Autodesk Fusion 360 part; units mm, degrees
(part 2 of 5)
sketch "Clamp Features" plane through (0, 0, 0) normal (0, 0, 1) x (1, 0, 0) in component "SpoilBoard"
  line L0 (576.58, 93.1525) -> (642.62, 93.1525)
  arc A0 (642.62, 93.1525) -> (642.62, 133.1525) centre (642.62, 113.1525) ccw
  line L1 (642.62, 133.1525) -> (576.58, 133.1525)
  arc A1 (576.58, 133.1525) -> (576.58, 93.1525) centre (576.58, 113.1525) ccw
  line L2 (576.58, 113.1525) -> (642.62, 113.1525) construction
  line L3 (0, 0) -> (1219.2, 0)
  line L4 (609.6, 0) -> (609.6, 113.1525)
  line L5 (33.02, 93.1525) -> (99.06, 93.1525)
  line L6 (99.06, 133.1525) -> (33.02, 133.1525)
  line L7 (33.02, 113.1525) -> (99.06, 113.1525) construction
  arc A2 (99.06, 93.1525) -> (99.06, 133.1525) centre (99.06, 113.1525) ccw
  arc A3 (33.02, 133.1525) -> (33.02, 93.1525) centre (33.02, 113.1525) ccw
  line L8 (214.2067, 93.1525) -> (280.2467, 93.1525)
  line L9 (280.2467, 133.1525) -> (214.2067, 133.1525)
  line L10 (214.2067, 113.1525) -> (280.2467, 113.1525) construction
  arc A4 (280.2467, 93.1525) -> (280.2467, 133.1525) centre (280.2467, 113.1525) ccw
  arc A5 (214.2067, 133.1525) -> (214.2067, 93.1525) centre (214.2067, 113.1525) ccw
  line L11 (395.3933, 93.1525) -> (461.4333, 93.1525)
  line L12 (461.4333, 133.1525) -> (395.3933, 133.1525)
  line L13 (395.3933, 113.1525) -> (461.4333, 113.1525) construction
  arc A6 (461.4333, 93.1525) -> (461.4333, 133.1525) centre (461.4333, 113.1525) ccw
  arc A7 (395.3933, 133.1525) -> (395.3933, 93.1525) centre (395.3933, 113.1525) ccw
  line L14 (757.7667, 93.1525) -> (823.8067, 93.1525)
  line L15 (823.8067, 133.1525) -> (757.7667, 133.1525)
  line L16 (757.7667, 113.1525) -> (823.8067, 113.1525) construction
  arc A8 (823.8067, 93.1525) -> (823.8067, 133.1525) centre (823.8067, 113.1525) ccw
  arc A9 (757.7667, 133.1525) -> (757.7667, 93.1525) centre (757.7667, 113.1525) ccw
  line L17 (938.9533, 93.1525) -> (1004.9933, 93.1525)
  line L18 (1004.9933, 133.1525) -> (938.9533, 133.1525)
  line L19 (938.9533, 113.1525) -> (1004.9933, 113.1525) construction
  arc A10 (1004.9933, 93.1525) -> (1004.9933, 133.1525) centre (1004.9933, 113.1525) ccw
  arc A11 (938.9533, 133.1525) -> (938.9533, 93.1525) centre (938.9533, 113.1525) ccw
  line L20 (1120.14, 93.1525) -> (1186.18, 93.1525)
  line L21 (1186.18, 133.1525) -> (1120.14, 133.1525)
  line L22 (1120.14, 113.1525) -> (1186.18, 113.1525) construction
  arc A12 (1186.18, 93.1525) -> (1186.18, 133.1525) centre (1186.18, 113.1525) ccw
  arc A13 (1120.14, 133.1525) -> (1120.14, 93.1525) centre (1120.14, 113.1525) ccw
  line L23 (33.02, 313.1525) -> (99.06, 313.1525)
  line L24 (99.06, 353.1525) -> (33.02, 353.1525)
  line L25 (33.02, 333.1525) -> (99.06, 333.1525) construction
  arc A14 (99.06, 313.1525) -> (99.06, 353.1525) centre (99.06, 333.1525) ccw
  arc A15 (33.02, 353.1525) -> (33.02, 313.1525) centre (33.02, 333.1525) ccw
  line L26 (214.2067, 313.1525) -> (280.2467, 313.1525)
  line L27 (280.2467, 353.1525) -> (214.2067, 353.1525)
  line L28 (214.2067, 333.1525) -> (280.2467, 333.1525) construction
  arc A16 (280.2467, 313.1525) -> (280.2467, 353.1525) centre (280.2467, 333.1525) ccw
  arc A17 (214.2067, 353.1525) -> (214.2067, 313.1525) centre (214.2067, 333.1525) ccw
  line L29 (395.3933, 313.1525) -> (461.4333, 313.1525)
  line L30 (461.4333, 353.1525) -> (395.3933, 353.1525)
  line L31 (395.3933, 333.1525) -> (461.4333, 333.1525) construction
  arc A18 (461.4333, 313.1525) -> (461.4333, 353.1525) centre (461.4333, 333.1525) ccw
  arc A19 (395.3933, 353.1525) -> (395.3933, 313.1525) centre (395.3933, 333.1525) ccw
  line L32 (576.58, 313.1525) -> (642.62, 313.1525)
  line L33 (642.62, 353.1525) -> (576.58, 353.1525)
  line L34 (576.58, 333.1525) -> (642.62, 333.1525) construction
  arc A20 (642.62, 313.1525) -> (642.62, 353.1525) centre (642.62, 333.1525) ccw
  arc A21 (576.58, 353.1525) -> (576.58, 313.1525) centre (576.58, 333.1525) ccw
  line L35 (757.7667, 313.1525) -> (823.8067, 313.1525)
  line L36 (823.8067, 353.1525) -> (757.7667, 353.1525)
  line L37 (757.7667, 333.1525) -> (823.8067, 333.1525) construction
  arc A22 (823.8067, 313.1525) -> (823.8067, 353.1525) centre (823.8067, 333.1525) ccw
  arc A23 (757.7667, 353.1525) -> (757.7667, 313.1525) centre (757.7667, 333.1525) ccw
  line L38 (938.9533, 313.1525) -> (1004.9933, 313.1525)
  line L39 (1004.9933, 353.1525) -> (938.9533, 353.1525)
  line L40 (938.9533, 333.1525) -> (1004.9933, 333.1525) construction
  arc A24 (1004.9933, 313.1525) -> (1004.9933, 353.1525) centre (1004.9933, 333.1525) ccw
  arc A25 (938.9533, 353.1525) -> (938.9533, 313.1525) centre (938.9533, 333.1525) ccw
  line L41 (1120.14, 313.1525) -> (1186.18, 313.1525)
  line L42 (1186.18, 353.1525) -> (1120.14, 353.1525)
  line L43 (1120.14, 333.1525) -> (1186.18, 333.1525) construction
  arc A26 (1186.18, 313.1525) -> (1186.18, 353.1525) centre (1186.18, 333.1525) ccw
  arc A27 (1120.14, 353.1525) -> (1120.14, 313.1525) centre (1120.14, 333.1525) ccw
  line L44 (665.5361, 207.1642) -> (731.5761, 207.1637)
  arc A28 (731.5761, 207.1637) -> (731.5763, 247.1637) centre (731.5762, 227.1637) ccw
  line L45 (665.5362, 227.1642) -> (731.5762, 227.1637) construction
  arc A29 (666.0507, 247.1575) -> (665.5361, 207.1642) centre (666.0526, 227.1575) ccw
  line L46 (731.5763, 247.1637) -> (666.0507, 247.1575)
  line L47 (666.0526, 227.1575) -> (731.1, 227.1575) construction
  line L48 (487.6237, 247.1637) -> (553.1493, 247.1575)
  arc A30 (553.6639, 207.1642) -> (553.1493, 247.1575) centre (553.1474, 227.1575) ccw
  line L49 (553.6639, 207.1642) -> (487.6239, 207.1637)
  arc A31 (487.6237, 247.1637) -> (487.6239, 207.1637) centre (487.6238, 227.1637) ccw
  line L50 (553.6638, 227.1642) -> (487.6238, 227.1637) construction
  line L51 (851.0526, 227.1575) -> (916.1, 227.1575) construction
  arc A32 (851.0507, 247.1575) -> (850.5361, 207.1642) centre (851.0526, 227.1575) ccw
  line L52 (850.5361, 207.1642) -> (916.5761, 207.1637)
  line L53 (916.5763, 247.1637) -> (851.0507, 247.1575)
  arc A33 (916.5761, 207.1637) -> (916.5763, 247.1637) centre (916.5762, 227.1637) ccw
  line L54 (850.5362, 227.1642) -> (916.5762, 227.1637) construction
  line L55 (1036.0526, 227.1575) -> (1101.1, 227.1575) construction
  arc A34 (1036.0507, 247.1575) -> (1035.5361, 207.1642) centre (1036.0526, 227.1575) ccw
  line L56 (1035.5361, 207.1642) -> (1101.5761, 207.1637)
  line L57 (1101.5763, 247.1637) -> (1036.0507, 247.1575)
  arc A35 (1101.5761, 207.1637) -> (1101.5763, 247.1637) centre (1101.5762, 227.1637) ccw
  line L58 (1035.5362, 227.1642) -> (1101.5762, 227.1637) construction
  line L59 (368.6639, 207.1642) -> (302.6239, 207.1637)
  arc A36 (368.6639, 207.1642) -> (368.1493, 247.1575) centre (368.1474, 227.1575) ccw
  line L60 (302.6237, 247.1637) -> (368.1493, 247.1575)
  arc A37 (302.6237, 247.1637) -> (302.6239, 207.1637) centre (302.6238, 227.1637) ccw
  line L61 (183.6639, 207.1642) -> (117.6239, 207.1637)
  arc A38 (183.6639, 207.1642) -> (183.1493, 247.1575) centre (183.1474, 227.1575) ccw
  line L62 (117.6237, 247.1637) -> (183.1493, 247.1575)
  arc A39 (117.6237, 247.1637) -> (117.6239, 207.1637) centre (117.6238, 227.1637) ccw
  line L63 (33.02, 713.1525) -> (99.06, 713.1525)
  arc A40 (461.4333, 713.1525) -> (461.4333, 753.1525) centre (461.4333, 733.1525) ccw
  arc A41 (395.3933, 753.1525) -> (395.3933, 713.1525) centre (395.3933, 733.1525) ccw
  line L64 (99.06, 753.1525) -> (33.02, 753.1525)
  arc A42 (576.58, 753.1525) -> (576.58, 713.1525) centre (576.58, 733.1525) ccw
  line L65 (33.02, 733.1525) -> (99.06, 733.1525) construction
  line L66 (214.2067, 713.1525) -> (280.2467, 713.1525)
  arc A43 (214.2067, 753.1525) -> (214.2067, 713.1525) centre (214.2067, 733.1525) ccw
  arc A44 (280.2467, 713.1525) -> (280.2467, 753.1525) centre (280.2467, 733.1525) ccw
  line L67 (280.2467, 753.1525) -> (214.2067, 753.1525)
  arc A45 (1120.14, 753.1525) -> (1120.14, 713.1525) centre (1120.14, 733.1525) ccw
  line L68 (938.9533, 733.1525) -> (1004.9933, 733.1525) construction
  line L69 (1120.14, 713.1525) -> (1186.18, 713.1525)
  line L70 (1186.18, 753.1525) -> (1120.14, 753.1525)
  line L71 (1120.14, 733.1525) -> (1186.18, 733.1525) construction
  arc A46 (1004.9933, 713.1525) -> (1004.9933, 753.1525) centre (1004.9933, 733.1525) ccw
  arc A47 (1186.18, 713.1525) -> (1186.18, 753.1525) centre (1186.18, 733.1525) ccw
  arc A48 (33.02, 753.1525) -> (33.02, 713.1525) centre (33.02, 733.1525) ccw
  line L72 (214.2067, 733.1525) -> (280.2467, 733.1525) construction
  arc A49 (99.06, 713.1525) -> (99.06, 753.1525) centre (99.06, 733.1525) ccw
  arc A50 (642.62, 713.1525) -> (642.62, 753.1525) centre (642.62, 733.1525) ccw
  arc A51 (823.8067, 713.1525) -> (823.8067, 753.1525) centre (823.8067, 733.1525) ccw
  arc A52 (938.9533, 753.1525) -> (938.9533, 713.1525) centre (938.9533, 733.1525) ccw
  line L73 (938.9533, 713.1525) -> (1004.9933, 713.1525)
  line L74 (1004.9933, 753.1525) -> (938.9533, 753.1525)
  line L75 (757.7667, 713.1525) -> (823.8067, 713.1525)
  line L76 (823.8067, 753.1525) -> (757.7667, 753.1525)
  line L77 (757.7667, 733.1525) -> (823.8067, 733.1525) construction
  arc A53 (757.7667, 753.1525) -> (757.7667, 713.1525) centre (757.7667, 733.1525) ccw
  line L78 (395.3933, 713.1525) -> (461.4333, 713.1525)
  line L79 (461.4333, 753.1525) -> (395.3933, 753.1525)
  line L80 (395.3933, 733.1525) -> (461.4333, 733.1525) construction
  line L81 (576.58, 713.1525) -> (642.62, 713.1525)
  line L82 (642.62, 753.1525) -> (576.58, 753.1525)
  line L83 (576.58, 733.1525) -> (642.62, 733.1525) construction
  line L84 (665.5361, 607.1642) -> (731.5761, 607.1637)
  line L85 (666.0526, 627.1575) -> (731.1, 627.1575) construction
  line L86 (850.5361, 607.1642) -> (916.5761, 607.1637)
  line L87 (665.5362, 627.1642) -> (731.5762, 627.1637) construction
  arc A54 (851.0507, 647.1575) -> (850.5361, 607.1642) centre (851.0526, 627.1575) ccw
  line L88 (850.5362, 627.1642) -> (916.5762, 627.1637) construction
  line L89 (851.0526, 627.1575) -> (916.1, 627.1575) construction
  arc A55 (916.5761, 607.1637) -> (916.5763, 647.1637) centre (916.5762, 627.1637) ccw
  line L90 (916.5763, 647.1637) -> (851.0507, 647.1575)
  line L91 (731.5763, 647.1637) -> (666.0507, 647.1575)
  arc A56 (731.5761, 607.1637) -> (731.5763, 647.1637) centre (731.5762, 627.1637) ccw
  arc A57 (1101.5761, 607.1637) -> (1101.5763, 647.1637) centre (1101.5762, 627.1637) ccw
  arc A58 (368.6639, 607.1642) -> (368.1493, 647.1575) centre (368.1474, 627.1575) ccw
  line L92 (368.6639, 607.1642) -> (302.6239, 607.1637)
  line L93 (302.6237, 647.1637) -> (368.1493, 647.1575)
  line L94 (183.6639, 607.1642) -> (117.6239, 607.1637)
  line L95 (117.6237, 647.1637) -> (183.1493, 647.1575)
  arc A59 (302.6237, 647.1637) -> (302.6239, 607.1637) centre (302.6238, 627.1637) ccw
  arc A60 (183.6639, 607.1642) -> (183.1493, 647.1575) centre (183.1474, 627.1575) ccw
  arc A61 (117.6237, 647.1637) -> (117.6239, 607.1637) centre (117.6238, 627.1637) ccw
  line L96 (1035.5361, 607.1642) -> (1101.5761, 607.1637)
  line L97 (1101.5763, 647.1637) -> (1036.0507, 647.1575)
  line L98 (1035.5362, 627.1642) -> (1101.5762, 627.1637) construction
  arc A62 (1036.0507, 647.1575) -> (1035.5361, 607.1642) centre (1036.0526, 627.1575) ccw
  arc A63 (553.6639, 607.1642) -> (553.1493, 647.1575) centre (553.1474, 627.1575) ccw
  line L99 (553.6638, 627.1642) -> (487.6238, 627.1637) construction
  line L100 (553.6639, 607.1642) -> (487.6239, 607.1637)
  line L101 (487.6237, 647.1637) -> (553.1493, 647.1575)
  arc A64 (487.6237, 647.1637) -> (487.6239, 607.1637) centre (487.6238, 627.1637) ccw
  line L102 (1036.0526, 627.1575) -> (1101.1, 627.1575) construction
  arc A65 (666.0507, 647.1575) -> (665.5361, 607.1642) centre (666.0526, 627.1575) ccw
  line L103 (938.9533, 493.1525) -> (1004.9933, 493.1525)
  line L104 (1004.9933, 533.1525) -> (938.9533, 533.1525)
  line L105 (938.9533, 513.1525) -> (1004.9933, 513.1525) construction
  line L106 (1120.14, 493.1525) -> (1186.18, 493.1525)
  line L107 (1186.18, 533.1525) -> (1120.14, 533.1525)
  line L108 (1120.14, 513.1525) -> (1186.18, 513.1525) construction
  arc A66 (1004.9933, 493.1525) -> (1004.9933, 533.1525) centre (1004.9933, 513.1525) ccw
  arc A67 (1186.18, 493.1525) -> (1186.18, 533.1525) centre (1186.18, 513.1525) ccw
  arc A68 (1120.14, 533.1525) -> (1120.14, 493.1525) centre (1120.14, 513.1525) ccw
  line L109 (757.7667, 493.1525) -> (823.8067, 493.1525)
  line L110 (757.7667, 513.1525) -> (823.8067, 513.1525) construction
  line L111 (823.8067, 533.1525) -> (757.7667, 533.1525)
  arc A69 (823.8067, 493.1525) -> (823.8067, 533.1525) centre (823.8067, 513.1525) ccw
  arc A70 (938.9533, 533.1525) -> (938.9533, 493.1525) centre (938.9533, 513.1525) ccw
  arc A71 (642.62, 493.1525) -> (642.62, 533.1525) centre (642.62, 513.1525) ccw
  line L112 (33.02, 493.1525) -> (99.06, 493.1525)
  arc A72 (576.58, 533.1525) -> (576.58, 493.1525) centre (576.58, 513.1525) ccw
  line L113 (99.06, 533.1525) -> (33.02, 533.1525)
  arc A73 (33.02, 533.1525) -> (33.02, 493.1525) centre (33.02, 513.1525) ccw
  arc A74 (461.4333, 493.1525) -> (461.4333, 533.1525) centre (461.4333, 513.1525) ccw
  line L114 (33.02, 513.1525) -> (99.06, 513.1525) construction
  arc A75 (99.06, 493.1525) -> (99.06, 533.1525) centre (99.06, 513.1525) ccw
  arc A76 (395.3933, 533.1525) -> (395.3933, 493.1525) centre (395.3933, 513.1525) ccw
  line L115 (214.2067, 493.1525) -> (280.2467, 493.1525)
  line L116 (280.2467, 533.1525) -> (214.2067, 533.1525)
  line L117 (214.2067, 513.1525) -> (280.2467, 513.1525) construction
  arc A77 (757.7667, 533.1525) -> (757.7667, 493.1525) centre (757.7667, 513.1525) ccw
  arc A78 (214.2067, 533.1525) -> (214.2067, 493.1525) centre (214.2067, 513.1525) ccw
  line L118 (576.58, 493.1525) -> (642.62, 493.1525)
  line L119 (576.58, 513.1525) -> (642.62, 513.1525) construction
  line L120 (609.6, 400) -> (609.6, 513.1525)
  line L121 (395.3933, 493.1525) -> (461.4333, 493.1525)
  line L122 (395.3933, 513.1525) -> (461.4333, 513.1525) construction
  arc A79 (280.2467, 493.1525) -> (280.2467, 533.1525) centre (280.2467, 513.1525) ccw
  line L123 (461.4333, 533.1525) -> (395.3933, 533.1525)
  line L124 (642.62, 533.1525) -> (576.58, 533.1525)
  line L125 (33.02, 1113.1525) -> (99.06, 1113.1525)
  arc A80 (461.4333, 1113.1525) -> (461.4333, 1153.1525) centre (461.4333, 1133.1525) ccw
  arc A81 (395.3933, 1153.1525) -> (395.3933, 1113.1525) centre (395.3933, 1133.1525) ccw
  line L126 (99.06, 1153.1525) -> (33.02, 1153.1525)
  arc A82 (576.58, 1153.1525) -> (576.58, 1113.1525) centre (576.58, 1133.1525) ccw
  line L127 (33.02, 1133.1525) -> (99.06, 1133.1525) construction
  line L128 (214.2067, 1113.1525) -> (280.2467, 1113.1525)
  arc A83 (214.2067, 1153.1525) -> (214.2067, 1113.1525) centre (214.2067, 1133.1525) ccw
  arc A84 (280.2467, 1113.1525) -> (280.2467, 1153.1525) centre (280.2467, 1133.1525) ccw
  line L129 (280.2467, 1153.1525) -> (214.2067, 1153.1525)
  arc A85 (1120.14, 1153.1525) -> (1120.14, 1113.1525) centre (1120.14, 1133.1525) ccw
  line L130 (938.9533, 1133.1525) -> (1004.9933, 1133.1525) construction
  line L131 (1120.14, 1113.1525) -> (1186.18, 1113.1525)
  line L132 (1186.18, 1153.1525) -> (1120.14, 1153.1525)
  line L133 (1120.14, 1133.1525) -> (1186.18, 1133.1525) construction
  arc A86 (1004.9933, 1113.1525) -> (1004.9933, 1153.1525) centre (1004.9933, 1133.1525) ccw
  arc A87 (1186.18, 1113.1525) -> (1186.18, 1153.1525) centre (1186.18, 1133.1525) ccw
  arc A88 (33.02, 1153.1525) -> (33.02, 1113.1525) centre (33.02, 1133.1525) ccw
  line L134 (214.2067, 1133.1525) -> (280.2467, 1133.1525) construction
  arc A89 (99.06, 1113.1525) -> (99.06, 1153.1525) centre (99.06, 1133.1525) ccw
  arc A90 (642.62, 1113.1525) -> (642.62, 1153.1525) centre (642.62, 1133.1525) ccw
  arc A91 (823.8067, 1113.1525) -> (823.8067, 1153.1525) centre (823.8067, 1133.1525) ccw
  arc A92 (938.9533, 1153.1525) -> (938.9533, 1113.1525) centre (938.9533, 1133.1525) ccw
  line L135 (938.9533, 1113.1525) -> (1004.9933, 1113.1525)
  line L136 (1004.9933, 1153.1525) -> (938.9533, 1153.1525)
  line L137 (757.7667, 1113.1525) -> (823.8067, 1113.1525)
  line L138 (823.8067, 1153.1525) -> (757.7667, 1153.1525)
  line L139 (757.7667, 1133.1525) -> (823.8067, 1133.1525) construction
  arc A93 (757.7667, 1153.1525) -> (757.7667, 1113.1525) centre (757.7667, 1133.1525) ccw
  line L140 (395.3933, 1113.1525) -> (461.4333, 1113.1525)
  line L141 (461.4333, 1153.1525) -> (395.3933, 1153.1525)
  line L142 (395.3933, 1133.1525) -> (461.4333, 1133.1525) construction
  line L143 (576.58, 1113.1525) -> (642.62, 1113.1525)
  line L144 (642.62, 1153.1525) -> (576.58, 1153.1525)
  line L145 (576.58, 1133.1525) -> (642.62, 1133.1525) construction
  line L146 (665.5361, 1007.1642) -> (731.5761, 1007.1637)
  line L147 (666.0526, 1027.1575) -> (731.1, 1027.1575) construction
  line L148 (850.5361, 1007.1642) -> (916.5761, 1007.1637)
  line L149 (665.5362, 1027.1642) -> (731.5762, 1027.1637) construction
  arc A94 (851.0507, 1047.1575) -> (850.5361, 1007.1642) centre (851.0526, 1027.1575) ccw
  line L150 (850.5362, 1027.1642) -> (916.5762, 1027.1637) construction
  line L151 (851.0526, 1027.1575) -> (916.1, 1027.1575) construction
  arc A95 (916.5761, 1007.1637) -> (916.5763, 1047.1637) centre (916.5762, 1027.1637) ccw
  line L152 (916.5763, 1047.1637) -> (851.0507, 1047.1575)
  line L153 (731.5763, 1047.1637) -> (666.0507, 1047.1575)
  arc A96 (731.5761, 1007.1637) -> (731.5763, 1047.1637) centre (731.5762, 1027.1637) ccw
  arc A97 (1101.5761, 1007.1637) -> (1101.5763, 1047.1637) centre (1101.5762, 1027.1637) ccw
  arc A98 (368.6639, 1007.1642) -> (368.1493, 1047.1575) centre (368.1474, 1027.1575) ccw
  line L154 (368.6639, 1007.1642) -> (302.6239, 1007.1637)
  line L155 (302.6237, 1047.1637) -> (368.1493, 1047.1575)
  line L156 (183.6639, 1007.1642) -> (117.6239, 1007.1637)
  line L157 (117.6237, 1047.1637) -> (183.1493, 1047.1575)
  arc A99 (302.6237, 1047.1637) -> (302.6239, 1007.1637) centre (302.6238, 1027.1637) ccw
  arc A100 (183.6639, 1007.1642) -> (183.1493, 1047.1575) centre (183.1474, 1027.1575) ccw
  arc A101 (117.6237, 1047.1637) -> (117.6239, 1007.1637) centre (117.6238, 1027.1637) ccw
  line L158 (1035.5361, 1007.1642) -> (1101.5761, 1007.1637)
  line L159 (1101.5763, 1047.1637) -> (1036.0507, 1047.1575)
  line L160 (1035.5362, 1027.1642) -> (1101.5762, 1027.1637) construction
  arc A102 (1036.0507, 1047.1575) -> (1035.5361, 1007.1642) centre (1036.0526, 1027.1575) ccw
  arc A103 (553.6639, 1007.1642) -> (553.1493, 1047.1575) centre (553.1474, 1027.1575) ccw
  line L161 (553.6638, 1027.1642) -> (487.6238, 1027.1637) construction
  line L162 (553.6639, 1007.1642) -> (487.6239, 1007.1637)
  line L163 (487.6237, 1047.1637) -> (553.1493, 1047.1575)
  arc A104 (487.6237, 1047.1637) -> (487.6239, 1007.1637) centre (487.6238, 1027.1637) ccw
  line L164 (1036.0526, 1027.1575) -> (1101.1, 1027.1575) construction
  arc A105 (666.0507, 1047.1575) -> (665.5361, 1007.1642) centre (666.0526, 1027.1575) ccw
  line L165 (938.9533, 893.1525) -> (1004.9933, 893.1525)
  line L166 (1004.9933, 933.1525) -> (938.9533, 933.1525)
  line L167 (938.9533, 913.1525) -> (1004.9933, 913.1525) construction
  line L168 (1120.14, 893.1525) -> (1186.18, 893.1525)
  line L169 (1186.18, 933.1525) -> (1120.14, 933.1525)
  line L170 (1120.14, 913.1525) -> (1186.18, 913.1525) construction
  arc A106 (1004.9933, 893.1525) -> (1004.9933, 933.1525) centre (1004.9933, 913.1525) ccw
  arc A107 (1186.18, 893.1525) -> (1186.18, 933.1525) centre (1186.18, 913.1525) ccw
  arc A108 (1120.14, 933.1525) -> (1120.14, 893.1525) centre (1120.14, 913.1525) ccw
  line L171 (757.7667, 893.1525) -> (823.8067, 893.1525)
  line L172 (757.7667, 913.1525) -> (823.8067, 913.1525) construction
  line L173 (823.8067, 933.1525) -> (757.7667, 933.1525)
  arc A109 (823.8067, 893.1525) -> (823.8067, 933.1525) centre (823.8067, 913.1525) ccw
  arc A110 (938.9533, 933.1525) -> (938.9533, 893.1525) centre (938.9533, 913.1525) ccw
  arc A111 (642.62, 893.1525) -> (642.62, 933.1525) centre (642.62, 913.1525) ccw
  line L174 (33.02, 893.1525) -> (99.06, 893.1525)
  arc A112 (576.58, 933.1525) -> (576.58, 893.1525) centre (576.58, 913.1525) ccw
  line L175 (99.06, 933.1525) -> (33.02, 933.1525)
  arc A113 (33.02, 933.1525) -> (33.02, 893.1525) centre (33.02, 913.1525) ccw
  arc A114 (461.4333, 893.1525) -> (461.4333, 933.1525) centre (461.4333, 913.1525) ccw
  line L176 (33.02, 913.1525) -> (99.06, 913.1525) construction
  arc A115 (99.06, 893.1525) -> (99.06, 933.1525) centre (99.06, 913.1525) ccw
  arc A116 (395.3933, 933.1525) -> (395.3933, 893.1525) centre (395.3933, 913.1525) ccw
  line L177 (214.2067, 893.1525) -> (280.2467, 893.1525)
  line L178 (280.2467, 933.1525) -> (214.2067, 933.1525)
  line L179 (214.2067, 913.1525) -> (280.2467, 913.1525) construction
  arc A117 (757.7667, 933.1525) -> (757.7667, 893.1525) centre (757.7667, 913.1525) ccw
  arc A118 (214.2067, 933.1525) -> (214.2067, 893.1525) centre (214.2067, 913.1525) ccw
  line L180 (576.58, 893.1525) -> (642.62, 893.1525)
  line L181 (576.58, 913.1525) -> (642.62, 913.1525) construction
  line L182 (609.6, 800) -> (609.6, 913.1525)
  line L183 (395.3933, 893.1525) -> (461.4333, 893.1525)
  line L184 (395.3933, 913.1525) -> (461.4333, 913.1525) construction
  arc A119 (280.2467, 893.1525) -> (280.2467, 933.1525) centre (280.2467, 913.1525) ccw
  line L185 (461.4333, 933.1525) -> (395.3933, 933.1525)
  line L186 (642.62, 933.1525) -> (576.58, 933.1525)
  line L187 (33.02, 1513.1525) -> (99.06, 1513.1525)
  arc A120 (461.4333, 1513.1525) -> (461.4333, 1553.1525) centre (461.4333, 1533.1525) ccw
  arc A121 (395.3933, 1553.1525) -> (395.3933, 1513.1525) centre (395.3933, 1533.1525) ccw
  line L188 (99.06, 1553.1525) -> (33.02, 1553.1525)
  arc A122 (576.58, 1553.1525) -> (576.58, 1513.1525) centre (576.58, 1533.1525) ccw
  line L189 (33.02, 1533.1525) -> (99.06, 1533.1525) construction
  line L190 (214.2067, 1513.1525) -> (280.2467, 1513.1525)
  arc A123 (214.2067, 1553.1525) -> (214.2067, 1513.1525) centre (214.2067, 1533.1525) ccw
  arc A124 (280.2467, 1513.1525) -> (280.2467, 1553.1525) centre (280.2467, 1533.1525) ccw
  line L191 (280.2467, 1553.1525) -> (214.2067, 1553.1525)
  arc A125 (1120.14, 1553.1525) -> (1120.14, 1513.1525) centre (1120.14, 1533.1525) ccw
  line L192 (938.9533, 1533.1525) -> (1004.9933, 1533.1525) construction
  line L193 (1120.14, 1513.1525) -> (1186.18, 1513.1525)
  line L194 (1186.18, 1553.1525) -> (1120.14, 1553.1525)
  line L195 (1120.14, 1533.1525) -> (1186.18, 1533.1525) construction
  arc A126 (1004.9933, 1513.1525) -> (1004.9933, 1553.1525) centre (1004.9933, 1533.1525) ccw
  arc A127 (1186.18, 1513.1525) -> (1186.18, 1553.1525) centre (1186.18, 1533.1525) ccw
  arc A128 (33.02, 1553.1525) -> (33.02, 1513.1525) centre (33.02, 1533.1525) ccw
  line L196 (214.2067, 1533.1525) -> (280.2467, 1533.1525) construction
  arc A129 (99.06, 1513.1525) -> (99.06, 1553.1525) centre (99.06, 1533.1525) ccw
  arc A130 (642.62, 1513.1525) -> (642.62, 1553.1525) centre (642.62, 1533.1525) ccw
  arc A131 (823.8067, 1513.1525) -> (823.8067, 1553.1525) centre (823.8067, 1533.1525) ccw
  arc A132 (938.9533, 1553.1525) -> (938.9533, 1513.1525) centre (938.9533, 1533.1525) ccw
  line L197 (938.9533, 1513.1525) -> (1004.9933, 1513.1525)
  line L198 (1004.9933, 1553.1525) -> (938.9533, 1553.1525)
  line L199 (757.7667, 1513.1525) -> (823.8067, 1513.1525)
  line L200 (823.8067, 1553.1525) -> (757.7667, 1553.1525)
  line L201 (757.7667, 1533.1525) -> (823.8067, 1533.1525) construction
  arc A133 (757.7667, 1553.1525) -> (757.7667, 1513.1525) centre (757.7667, 1533.1525) ccw
  line L202 (395.3933, 1513.1525) -> (461.4333, 1513.1525)
  line L203 (461.4333, 1553.1525) -> (395.3933, 1553.1525)
  line L204 (395.3933, 1533.1525) -> (461.4333, 1533.1525) construction
  line L205 (576.58, 1513.1525) -> (642.62, 1513.1525)
  line L206 (642.62, 1553.1525) -> (576.58, 1553.1525)
  line L207 (576.58, 1533.1525) -> (642.62, 1533.1525) construction
  line L208 (665.5361, 1407.1642) -> (731.5761, 1407.1637)
  line L209 (666.0526, 1427.1575) -> (731.1, 1427.1575) construction
  line L210 (850.5361, 1407.1642) -> (916.5761, 1407.1637)
  line L211 (665.5362, 1427.1642) -> (731.5762, 1427.1637) construction
  arc A134 (851.0507, 1447.1575) -> (850.5361, 1407.1642) centre (851.0526, 1427.1575) ccw
  line L212 (850.5362, 1427.1642) -> (916.5762, 1427.1637) construction
  line L213 (851.0526, 1427.1575) -> (916.1, 1427.1575) construction
  arc A135 (916.5761, 1407.1637) -> (916.5763, 1447.1637) centre (916.5762, 1427.1637) ccw
  line L214 (916.5763, 1447.1637) -> (851.0507, 1447.1575)
  line L215 (731.5763, 1447.1637) -> (666.0507, 1447.1575)
  arc A136 (731.5761, 1407.1637) -> (731.5763, 1447.1637) centre (731.5762, 1427.1637) ccw
  arc A137 (1101.5761, 1407.1637) -> (1101.5763, 1447.1637) centre (1101.5762, 1427.1637) ccw
  arc A138 (368.6639, 1407.1642) -> (368.1493, 1447.1575) centre (368.1474, 1427.1575) ccw
  line L216 (368.6639, 1407.1642) -> (302.6239, 1407.1637)
  line L217 (302.6237, 1447.1637) -> (368.1493, 1447.1575)
  line L218 (183.6639, 1407.1642) -> (117.6239, 1407.1637)
  line L219 (117.6237, 1447.1637) -> (183.1493, 1447.1575)
  arc A139 (302.6237, 1447.1637) -> (302.6239, 1407.1637) centre (302.6238, 1427.1637) ccw
  arc A140 (183.6639, 1407.1642) -> (183.1493, 1447.1575) centre (183.1474, 1427.1575) ccw
  arc A141 (117.6237, 1447.1637) -> (117.6239, 1407.1637) centre (117.6238, 1427.1637) ccw
  line L220 (1035.5361, 1407.1642) -> (1101.5761, 1407.1637)
  line L221 (1101.5763, 1447.1637) -> (1036.0507, 1447.1575)
  line L222 (1035.5362, 1427.1642) -> (1101.5762, 1427.1637) construction
  arc A142 (1036.0507, 1447.1575) -> (1035.5361, 1407.1642) centre (1036.0526, 1427.1575) ccw
  arc A143 (553.6639, 1407.1642) -> (553.1493, 1447.1575) centre (553.1474, 1427.1575) ccw
  line L223 (553.6638, 1427.1642) -> (487.6238, 1427.1637) construction
  line L224 (553.6639, 1407.1642) -> (487.6239, 1407.1637)
  line L225 (487.6237, 1447.1637) -> (553.1493, 1447.1575)
  arc A144 (487.6237, 1447.1637) -> (487.6239, 1407.1637) centre (487.6238, 1427.1637) ccw
  line L226 (1036.0526, 1427.1575) -> (1101.1, 1427.1575) construction
  arc A145 (666.0507, 1447.1575) -> (665.5361, 1407.1642) centre (666.0526, 1427.1575) ccw
  line L227 (938.9533, 1293.1525) -> (1004.9933, 1293.1525)
  line L228 (1004.9933, 1333.1525) -> (938.9533, 1333.1525)
  line L229 (938.9533, 1313.1525) -> (1004.9933, 1313.1525) construction
  line L230 (1120.14, 1293.1525) -> (1186.18, 1293.1525)
  line L231 (1186.18, 1333.1525) -> (1120.14, 1333.1525)
  line L232 (1120.14, 1313.1525) -> (1186.18, 1313.1525) construction
  arc A146 (1004.9933, 1293.1525) -> (1004.9933, 1333.1525) centre (1004.9933, 1313.1525) ccw
  arc A147 (1186.18, 1293.1525) -> (1186.18, 1333.1525) centre (1186.18, 1313.1525) ccw
  arc A148 (1120.14, 1333.1525) -> (1120.14, 1293.1525) centre (1120.14, 1313.1525) ccw
  line L233 (757.7667, 1293.1525) -> (823.8067, 1293.1525)
  line L234 (757.7667, 1313.1525) -> (823.8067, 1313.1525) construction
  line L235 (823.8067, 1333.1525) -> (757.7667, 1333.1525)
  arc A149 (823.8067, 1293.1525) -> (823.8067, 1333.1525) centre (823.8067, 1313.1525) ccw
  arc A150 (938.9533, 1333.1525) -> (938.9533, 1293.1525) centre (938.9533, 1313.1525) ccw
  arc A151 (642.62, 1293.1525) -> (642.62, 1333.1525) centre (642.62, 1313.1525) ccw
  line L236 (33.02, 1293.1525) -> (99.06, 1293.1525)
  arc A152 (576.58, 1333.1525) -> (576.58, 1293.1525) centre (576.58, 1313.1525) ccw
  line L237 (99.06, 1333.1525) -> (33.02, 1333.1525)
  arc A153 (33.02, 1333.1525) -> (33.02, 1293.1525) centre (33.02, 1313.1525) ccw
  arc A154 (461.4333, 1293.1525) -> (461.4333, 1333.1525) centre (461.4333, 1313.1525) ccw
  line L238 (33.02, 1313.1525) -> (99.06, 1313.1525) construction
  arc A155 (99.06, 1293.1525) -> (99.06, 1333.1525) centre (99.06, 1313.1525) ccw
  arc A156 (395.3933, 1333.1525) -> (395.3933, 1293.1525) centre (395.3933, 1313.1525) ccw
  line L239 (214.2067, 1293.1525) -> (280.2467, 1293.1525)
  line L240 (280.2467, 1333.1525) -> (214.2067, 1333.1525)
  line L241 (214.2067, 1313.1525) -> (280.2467, 1313.1525) construction
  arc A157 (757.7667, 1333.1525) -> (757.7667, 1293.1525) centre (757.7667, 1313.1525) ccw
  arc A158 (214.2067, 1333.1525) -> (214.2067, 1293.1525) centre (214.2067, 1313.1525) ccw
  line L242 (576.58, 1293.1525) -> (642.62, 1293.1525)
  line L243 (576.58, 1313.1525) -> (642.62, 1313.1525) construction
  line L244 (609.6, 1200) -> (609.6, 1313.1525)
  line L245 (395.3933, 1293.1525) -> (461.4333, 1293.1525)
  line L246 (395.3933, 1313.1525) -> (461.4333, 1313.1525) construction
  arc A159 (280.2467, 1293.1525) -> (280.2467, 1333.1525) centre (280.2467, 1313.1525) ccw
  line L247 (461.4333, 1333.1525) -> (395.3933, 1333.1525)
  line L248 (642.62, 1333.1525) -> (576.58, 1333.1525)
  line L249 (33.02, 1913.1525) -> (99.06, 1913.1525)
  arc A160 (461.4333, 1913.1525) -> (461.4333, 1953.1525) centre (461.4333, 1933.1525) ccw
  arc A161 (395.3933, 1953.1525) -> (395.3933, 1913.1525) centre (395.3933, 1933.1525) ccw
  line L250 (99.06, 1953.1525) -> (33.02, 1953.1525)
  arc A162 (576.58, 1953.1525) -> (576.58, 1913.1525) centre (576.58, 1933.1525) ccw
  line L251 (33.02, 1933.1525) -> (99.06, 1933.1525) construction
  line L252 (214.2067, 1913.1525) -> (280.2467, 1913.1525)
  arc A163 (214.2067, 1953.1525) -> (214.2067, 1913.1525) centre (214.2067, 1933.1525) ccw
  arc A164 (280.2467, 1913.1525) -> (280.2467, 1953.1525) centre (280.2467, 1933.1525) ccw
  line L253 (280.2467, 1953.1525) -> (214.2067, 1953.1525)
  arc A165 (1120.14, 1953.1525) -> (1120.14, 1913.1525) centre (1120.14, 1933.1525) ccw
  line L254 (938.9533, 1933.1525) -> (1004.9933, 1933.1525) construction
  line L255 (1120.14, 1913.1525) -> (1186.18, 1913.1525)
  line L256 (1186.18, 1953.1525) -> (1120.14, 1953.1525)
  line L257 (1120.14, 1933.1525) -> (1186.18, 1933.1525) construction
  arc A166 (1004.9933, 1913.1525) -> (1004.9933, 1953.1525) centre (1004.9933, 1933.1525) ccw
  arc A167 (1186.18, 1913.1525) -> (1186.18, 1953.1525) centre (1186.18, 1933.1525) ccw
  arc A168 (33.02, 1953.1525) -> (33.02, 1913.1525) centre (33.02, 1933.1525) ccw
  line L258 (214.2067, 1933.1525) -> (280.2467, 1933.1525) construction
  arc A169 (99.06, 1913.1525) -> (99.06, 1953.1525) centre (99.06, 1933.1525) ccw
  arc A170 (642.62, 1913.1525) -> (642.62, 1953.1525) centre (642.62, 1933.1525) ccw
  arc A171 (823.8067, 1913.1525) -> (823.8067, 1953.1525) centre (823.8067, 1933.1525) ccw
  arc A172 (938.9533, 1953.1525) -> (938.9533, 1913.1525) centre (938.9533, 1933.1525) ccw
  line L259 (938.9533, 1913.1525) -> (1004.9933, 1913.1525)
  line L260 (1004.9933, 1953.1525) -> (938.9533, 1953.1525)
  line L261 (757.7667, 1913.1525) -> (823.8067, 1913.1525)
  line L262 (823.8067, 1953.1525) -> (757.7667, 1953.1525)
  line L263 (757.7667, 1933.1525) -> (823.8067, 1933.1525) construction
  arc A173 (757.7667, 1953.1525) -> (757.7667, 1913.1525) centre (757.7667, 1933.1525) ccw
  line L264 (395.3933, 1913.1525) -> (461.4333, 1913.1525)
  line L265 (461.4333, 1953.1525) -> (395.3933, 1953.1525)
  line L266 (395.3933, 1933.1525) -> (461.4333, 1933.1525) construction
  line L267 (576.58, 1913.1525) -> (642.62, 1913.1525)
  line L268 (642.62, 1953.1525) -> (576.58, 1953.1525)
  line L269 (576.58, 1933.1525) -> (642.62, 1933.1525) construction
  line L270 (665.5361, 1807.1642) -> (731.5761, 1807.1637)
  line L271 (666.0526, 1827.1575) -> (731.1, 1827.1575) construction
  line L272 (850.5361, 1807.1642) -> (916.5761, 1807.1637)
  line L273 (665.5362, 1827.1642) -> (731.5762, 1827.1637) construction
  arc A174 (851.0507, 1847.1575) -> (850.5361, 1807.1642) centre (851.0526, 1827.1575) ccw
  line L274 (850.5362, 1827.1642) -> (916.5762, 1827.1637) construction
  line L275 (851.0526, 1827.1575) -> (916.1, 1827.1575) construction
  arc A175 (916.5761, 1807.1637) -> (916.5763, 1847.1637) centre (916.5762, 1827.1637) ccw
  line L276 (916.5763, 1847.1637) -> (851.0507, 1847.1575)
  line L277 (731.5763, 1847.1637) -> (666.0507, 1847.1575)
  arc A176 (731.5761, 1807.1637) -> (731.5763, 1847.1637) centre (731.5762, 1827.1637) ccw
  arc A177 (1101.5761, 1807.1637) -> (1101.5763, 1847.1637) centre (1101.5762, 1827.1637) ccw
  arc A178 (368.6639, 1807.1642) -> (368.1493, 1847.1575) centre (368.1474, 1827.1575) ccw
  line L278 (368.6639, 1807.1642) -> (302.6239, 1807.1637)
  line L279 (302.6237, 1847.1637) -> (368.1493, 1847.1575)
  line L280 (183.6639, 1807.1642) -> (117.6239, 1807.1637)
  line L281 (117.6237, 1847.1637) -> (183.1493, 1847.1575)
  arc A179 (302.6237, 1847.1637) -> (302.6239, 1807.1637) centre (302.6238, 1827.1637) ccw
  arc A180 (183.6639, 1807.1642) -> (183.1493, 1847.1575) centre (183.1474, 1827.1575) ccw
  arc A181 (117.6237, 1847.1637) -> (117.6239, 1807.1637) centre (117.6238, 1827.1637) ccw
  line L282 (1035.5361, 1807.1642) -> (1101.5761, 1807.1637)
  line L283 (1101.5763, 1847.1637) -> (1036.0507, 1847.1575)
  line L284 (1035.5362, 1827.1642) -> (1101.5762, 1827.1637) construction
  arc A182 (1036.0507, 1847.1575) -> (1035.5361, 1807.1642) centre (1036.0526, 1827.1575) ccw
  arc A183 (553.6639, 1807.1642) -> (553.1493, 1847.1575) centre (553.1474, 1827.1575) ccw
  line L285 (553.6638, 1827.1642) -> (487.6238, 1827.1637) construction
  line L286 (553.6639, 1807.1642) -> (487.6239, 1807.1637)
  line L287 (487.6237, 1847.1637) -> (553.1493, 1847.1575)
  arc A184 (487.6237, 1847.1637) -> (487.6239, 1807.1637) centre (487.6238, 1827.1637) ccw
  line L288 (1036.0526, 1827.1575) -> (1101.1, 1827.1575) construction
  arc A185 (666.0507, 1847.1575) -> (665.5361, 1807.1642) centre (666.0526, 1827.1575) ccw
  line L289 (938.9533, 1693.1525) -> (1004.9933, 1693.1525)
  line L290 (1004.9933, 1733.1525) -> (938.9533, 1733.1525)
  line L291 (938.9533, 1713.1525) -> (1004.9933, 1713.1525) construction
  line L292 (1120.14, 1693.1525) -> (1186.18, 1693.1525)
  line L293 (1186.18, 1733.1525) -> (1120.14, 1733.1525)
  line L294 (1120.14, 1713.1525) -> (1186.18, 1713.1525) construction
  arc A186 (1004.9933, 1693.1525) -> (1004.9933, 1733.1525) centre (1004.9933, 1713.1525) ccw
  arc A187 (1186.18, 1693.1525) -> (1186.18, 1733.1525) centre (1186.18, 1713.1525) ccw
  arc A188 (1120.14, 1733.1525) -> (1120.14, 1693.1525) centre (1120.14, 1713.1525) ccw
  line L295 (757.7667, 1693.1525) -> (823.8067, 1693.1525)
  line L296 (757.7667, 1713.1525) -> (823.8067, 1713.1525) construction
  line L297 (823.8067, 1733.1525) -> (757.7667, 1733.1525)
  arc A189 (823.8067, 1693.1525) -> (823.8067, 1733.1525) centre (823.8067, 1713.1525) ccw
  arc A190 (938.9533, 1733.1525) -> (938.9533, 1693.1525) centre (938.9533, 1713.1525) ccw
  arc A191 (642.62, 1693.1525) -> (642.62, 1733.1525) centre (642.62, 1713.1525) ccw
  line L298 (33.02, 1693.1525) -> (99.06, 1693.1525)
  arc A192 (576.58, 1733.1525) -> (576.58, 1693.1525) centre (576.58, 1713.1525) ccw
  line L299 (99.06, 1733.1525) -> (33.02, 1733.1525)
  arc A193 (33.02, 1733.1525) -> (33.02, 1693.1525) centre (33.02, 1713.1525) ccw
  arc A194 (461.4333, 1693.1525) -> (461.4333, 1733.1525) centre (461.4333, 1713.1525) ccw
  line L300 (33.02, 1713.1525) -> (99.06, 1713.1525) construction
  arc A195 (99.06, 1693.1525) -> (99.06, 1733.1525) centre (99.06, 1713.1525) ccw
  arc A196 (395.3933, 1733.1525) -> (395.3933, 1693.1525) centre (395.3933, 1713.1525) ccw
  line L301 (214.2067, 1693.1525) -> (280.2467, 1693.1525)
  line L302 (280.2467, 1733.1525) -> (214.2067, 1733.1525)
  line L303 (214.2067, 1713.1525) -> (280.2467, 1713.1525) construction
  arc A197 (757.7667, 1733.1525) -> (757.7667, 1693.1525) centre (757.7667, 1713.1525) ccw
  arc A198 (214.2067, 1733.1525) -> (214.2067, 1693.1525) centre (214.2067, 1713.1525) ccw
  line L304 (576.58, 1693.1525) -> (642.62, 1693.1525)
  line L305 (576.58, 1713.1525) -> (642.62, 1713.1525) construction
  line L306 (609.6, 1600) -> (609.6, 1713.1525)
  line L307 (395.3933, 1693.1525) -> (461.4333, 1693.1525)
  line L308 (395.3933, 1713.1525) -> (461.4333, 1713.1525) construction
  arc A199 (280.2467, 1693.1525) -> (280.2467, 1733.1525) centre (280.2467, 1713.1525) ccw
  line L309 (461.4333, 1733.1525) -> (395.3933, 1733.1525)
  line L310 (642.62, 1733.1525) -> (576.58, 1733.1525)
  line L311 (33.02, 2313.1525) -> (99.06, 2313.1525)
  arc A200 (461.4333, 2313.1525) -> (461.4333, 2353.1525) centre (461.4333, 2333.1525) ccw
  arc A201 (395.3933, 2353.1525) -> (395.3933, 2313.1525) centre (395.3933, 2333.1525) ccw
  line L312 (99.06, 2353.1525) -> (33.02, 2353.1525)
  arc A202 (576.58, 2353.1525) -> (576.58, 2313.1525) centre (576.58, 2333.1525) ccw
  line L313 (33.02, 2333.1525) -> (99.06, 2333.1525) construction
  line L314 (214.2067, 2313.1525) -> (280.2467, 2313.1525)
  arc A203 (214.2067, 2353.1525) -> (214.2067, 2313.1525) centre (214.2067, 2333.1525) ccw
  arc A204 (280.2467, 2313.1525) -> (280.2467, 2353.1525) centre (280.2467, 2333.1525) ccw
  line L315 (280.2467, 2353.1525) -> (214.2067, 2353.1525)
  arc A205 (1120.14, 2353.1525) -> (1120.14, 2313.1525) centre (1120.14, 2333.1525) ccw
  line L316 (938.9533, 2333.1525) -> (1004.9933, 2333.1525) construction
  line L317 (1120.14, 2313.1525) -> (1186.18, 2313.1525)
  line L318 (1186.18, 2353.1525) -> (1120.14, 2353.1525)
  line L319 (1120.14, 2333.1525) -> (1186.18, 2333.1525) construction
  arc A206 (1004.9933, 2313.1525) -> (1004.9933, 2353.1525) centre (1004.9933, 2333.1525) ccw
  arc A207 (1186.18, 2313.1525) -> (1186.18, 2353.1525) centre (1186.18, 2333.1525) ccw
  arc A208 (33.02, 2353.1525) -> (33.02, 2313.1525) centre (33.02, 2333.1525) ccw
  line L320 (214.2067, 2333.1525) -> (280.2467, 2333.1525) construction
  arc A209 (99.06, 2313.1525) -> (99.06, 2353.1525) centre (99.06, 2333.1525) ccw
  arc A210 (642.62, 2313.1525) -> (642.62, 2353.1525) centre (642.62, 2333.1525) ccw
  arc A211 (823.8067, 2313.1525) -> (823.8067, 2353.1525) centre (823.8067, 2333.1525) ccw
  arc A212 (938.9533, 2353.1525) -> (938.9533, 2313.1525) centre (938.9533, 2333.1525) ccw
  line L321 (938.9533, 2313.1525) -> (1004.9933, 2313.1525)
  line L322 (1004.9933, 2353.1525) -> (938.9533, 2353.1525)
  line L323 (757.7667, 2313.1525) -> (823.8067, 2313.1525)
  line L324 (823.8067, 2353.1525) -> (757.7667, 2353.1525)
  line L325 (757.7667, 2333.1525) -> (823.8067, 2333.1525) construction
  arc A213 (757.7667, 2353.1525) -> (757.7667, 2313.1525) centre (757.7667, 2333.1525) ccw
  line L326 (395.3933, 2313.1525) -> (461.4333, 2313.1525)
  line L327 (461.4333, 2353.1525) -> (395.3933, 2353.1525)
  line L328 (395.3933, 2333.1525) -> (461.4333, 2333.1525) construction
  line L329 (576.58, 2313.1525) -> (642.62, 2313.1525)
  line L330 (642.62, 2353.1525) -> (576.58, 2353.1525)
  line L331 (576.58, 2333.1525) -> (642.62, 2333.1525) construction
  line L332 (665.5361, 2207.1642) -> (731.5761, 2207.1637)
  line L333 (666.0526, 2227.1575) -> (731.1, 2227.1575) construction
  line L334 (850.5361, 2207.1642) -> (916.5761, 2207.1637)
  line L335 (665.5362, 2227.1642) -> (731.5762, 2227.1637) construction
  arc A214 (851.0507, 2247.1575) -> (850.5361, 2207.1642) centre (851.0526, 2227.1575) ccw
  line L336 (850.5362, 2227.1642) -> (916.5762, 2227.1637) construction
  line L337 (851.0526, 2227.1575) -> (916.1, 2227.1575) construction
  arc A215 (916.5761, 2207.1637) -> (916.5763, 2247.1637) centre (916.5762, 2227.1637) ccw
  line L338 (916.5763, 2247.1637) -> (851.0507, 2247.1575)
  line L339 (731.5763, 2247.1637) -> (666.0507, 2247.1575)
  arc A216 (731.5761, 2207.1637) -> (731.5763, 2247.1637) centre (731.5762, 2227.1637) ccw
  arc A217 (1101.5761, 2207.1637) -> (1101.5763, 2247.1637) centre (1101.5762, 2227.1637) ccw
  arc A218 (368.6639, 2207.1642) -> (368.1493, 2247.1575) centre (368.1474, 2227.1575) ccw
  line L340 (368.6639, 2207.1642) -> (302.6239, 2207.1637)
  line L341 (302.6237, 2247.1637) -> (368.1493, 2247.1575)
  line L342 (183.6639, 2207.1642) -> (117.6239, 2207.1637)
  line L343 (117.6237, 2247.1637) -> (183.1493, 2247.1575)
  arc A219 (302.6237, 2247.1637) -> (302.6239, 2207.1637) centre (302.6238, 2227.1637) ccw
  arc A220 (183.6639, 2207.1642) -> (183.1493, 2247.1575) centre (183.1474, 2227.1575) ccw
  arc A221 (117.6237, 2247.1637) -> (117.6239, 2207.1637) centre (117.6238, 2227.1637) ccw
  line L344 (1035.5361, 2207.1642) -> (1101.5761, 2207.1637)
  line L345 (1101.5763, 2247.1637) -> (1036.0507, 2247.1575)
  line L346 (1035.5362, 2227.1642) -> (1101.5762, 2227.1637) construction
  arc A222 (1036.0507, 2247.1575) -> (1035.5361, 2207.1642) centre (1036.0526, 2227.1575) ccw
  arc A223 (553.6639, 2207.1642) -> (553.1493, 2247.1575) centre (553.1474, 2227.1575) ccw
  line L347 (553.6638, 2227.1642) -> (487.6238, 2227.1637) construction
  line L348 (553.6639, 2207.1642) -> (487.6239, 2207.1637)
  line L349 (487.6237, 2247.1637) -> (553.1493, 2247.1575)
  arc A224 (487.6237, 2247.1637) -> (487.6239, 2207.1637) centre (487.6238, 2227.1637) ccw
  line L350 (1036.0526, 2227.1575) -> (1101.1, 2227.1575) construction
  arc A225 (666.0507, 2247.1575) -> (665.5361, 2207.1642) centre (666.0526, 2227.1575) ccw
  line L351 (938.9533, 2093.1525) -> (1004.9933, 2093.1525)
  line L352 (1004.9933, 2133.1525) -> (938.9533, 2133.1525)
  line L353 (938.9533, 2113.1525) -> (1004.9933, 2113.1525) construction
  line L354 (1120.14, 2093.1525) -> (1186.18, 2093.1525)
  line L355 (1186.18, 2133.1525) -> (1120.14, 2133.1525)
  line L356 (1120.14, 2113.1525) -> (1186.18, 2113.1525) construction
  arc A226 (1004.9933, 2093.1525) -> (1004.9933, 2133.1525) centre (1004.9933, 2113.1525) ccw
  arc A227 (1186.18, 2093.1525) -> (1186.18, 2133.1525) centre (1186.18, 2113.1525) ccw
  arc A228 (1120.14, 2133.1525) -> (1120.14, 2093.1525) centre (1120.14, 2113.1525) ccw
  line L357 (757.7667, 2093.1525) -> (823.8067, 2093.1525)
  line L358 (757.7667, 2113.1525) -> (823.8067, 2113.1525) construction
  line L359 (823.8067, 2133.1525) -> (757.7667, 2133.1525)
  arc A229 (823.8067, 2093.1525) -> (823.8067, 2133.1525) centre (823.8067, 2113.1525) ccw
  arc A230 (938.9533, 2133.1525) -> (938.9533, 2093.1525) centre (938.9533, 2113.1525) ccw
  arc A231 (642.62, 2093.1525) -> (642.62, 2133.1525) centre (642.62, 2113.1525) ccw
  line L360 (33.02, 2093.1525) -> (99.06, 2093.1525)
  arc A232 (576.58, 2133.1525) -> (576.58, 2093.1525) centre (576.58, 2113.1525) ccw
  line L361 (99.06, 2133.1525) -> (33.02, 2133.1525)
  arc A233 (33.02, 2133.1525) -> (33.02, 2093.1525) centre (33.02, 2113.1525) ccw
  arc A234 (461.4333, 2093.1525) -> (461.4333, 2133.1525) centre (461.4333, 2113.1525) ccw
  line L362 (33.02, 2113.1525) -> (99.06, 2113.1525) construction
  arc A235 (99.06, 2093.1525) -> (99.06, 2133.1525) centre (99.06, 2113.1525) ccw
  arc A236 (395.3933, 2133.1525) -> (395.3933, 2093.1525) centre (395.3933, 2113.1525) ccw
  line L363 (214.2067, 2093.1525) -> (280.2467, 2093.1525)
  line L364 (280.2467, 2133.1525) -> (214.2067, 2133.1525)
  line L365 (214.2067, 2113.1525) -> (280.2467, 2113.1525) construction
  arc A237 (757.7667, 2133.1525) -> (757.7667, 2093.1525) centre (757.7667, 2113.1525) ccw
  arc A238 (214.2067, 2133.1525) -> (214.2067, 2093.1525) centre (214.2067, 2113.1525) ccw
  line L366 (576.58, 2093.1525) -> (642.62, 2093.1525)
  line L367 (576.58, 2113.1525) -> (642.62, 2113.1525) construction
  line L368 (609.6, 2000) -> (609.6, 2113.1525)
  line L369 (395.3933, 2093.1525) -> (461.4333, 2093.1525)
  line L370 (395.3933, 2113.1525) -> (461.4333, 2113.1525) construction
  arc A239 (280.2467, 2093.1525) -> (280.2467, 2133.1525) centre (280.2467, 2113.1525) ccw
  line L371 (461.4333, 2133.1525) -> (395.3933, 2133.1525)
  line L372 (642.62, 2133.1525) -> (576.58, 2133.1525)
  point P0 (609.6, 0)
  point P1 (66.04, 113.1525)
  point P2 (247.2267, 113.1525)
  point P3 (428.4133, 113.1525)
  point P4 (790.7867, 113.1525)
  point P5 (971.9733, 113.1525)
  point P6 (1153.16, 113.1525)
  point P7 (66.04, 333.1525)
  point P8 (247.2267, 333.1525)
  point P9 (428.4133, 333.1525)
  point P10 (609.6, 333.1525)
  point P11 (790.7867, 333.1525)
  point P12 (971.9733, 333.1525)
  point P13 (1153.16, 333.1525)
  point P14 (66.04, 733.1525)
  point P15 (790.7867, 733.1525)
  point P16 (1153.16, 733.1525)
  point P17 (971.9733, 733.1525)
  point P18 (247.2267, 733.1525)
  point P19 (428.4133, 733.1525)
  point P20 (609.6, 733.1525)
  point P21 (247.2267, 513.1525)
  point P22 (1153.16, 513.1525)
  point P23 (428.4133, 513.1525)
  point P24 (971.9733, 513.1525)
  point P25 (790.7867, 513.1525)
  point P26 (66.04, 513.1525)
  point P27 (66.04, 1133.1525)
  point P28 (790.7867, 1133.1525)
  point P29 (1153.16, 1133.1525)
  point P30 (971.9733, 1133.1525)
  point P31 (247.2267, 1133.1525)
  point P32 (428.4133, 1133.1525)
  point P33 (609.6, 1133.1525)
  point P34 (247.2267, 913.1525)
  point P35 (1153.16, 913.1525)
  point P36 (428.4133, 913.1525)
  point P37 (971.9733, 913.1525)
  point P38 (790.7867, 913.1525)
  point P39 (66.04, 913.1525)
  point P40 (66.04, 1533.1525)
  point P41 (790.7867, 1533.1525)
  point P42 (1153.16, 1533.1525)
  point P43 (971.9733, 1533.1525)
  point P44 (247.2267, 1533.1525)
  point P45 (428.4133, 1533.1525)
  point P46 (609.6, 1533.1525)
  point P47 (247.2267, 1313.1525)
  point P48 (1153.16, 1313.1525)
  point P49 (428.4133, 1313.1525)
  point P50 (971.9733, 1313.1525)
  point P51 (790.7867, 1313.1525)
  point P52 (66.04, 1313.1525)
  point P53 (66.04, 1933.1525)
  point P54 (790.7867, 1933.1525)
  point P55 (1153.16, 1933.1525)
  point P56 (971.9733, 1933.1525)
  point P57 (247.2267, 1933.1525)
  point P58 (428.4133, 1933.1525)
  point P59 (609.6, 1933.1525)
  point P60 (247.2267, 1713.1525)
  point P61 (1153.16, 1713.1525)
  point P62 (428.4133, 1713.1525)
  point P63 (971.9733, 1713.1525)
  point P64 (790.7867, 1713.1525)
  point P65 (66.04, 1713.1525)
  point P66 (66.04, 2333.1525)
  point P67 (790.7867, 2333.1525)
  point P68 (1153.16, 2333.1525)
  point P69 (971.9733, 2333.1525)
  point P70 (247.2267, 2333.1525)
  point P71 (428.4133, 2333.1525)
  point P72 (609.6, 2333.1525)
  point P73 (247.2267, 2113.1525)
  point P74 (1153.16, 2113.1525)
  point P75 (428.4133, 2113.1525)
  point P76 (971.9733, 2113.1525)
  point P77 (790.7867, 2113.1525)
  point P78 (66.04, 2113.1525)
  dimension "d52" = 113.1525
  dimension "d56" = 20
  dimension "d58" = 66.04
  dimension "d61" = 543.56
  dimension "d62" = 220
  dimension "d64" = 66.04
  dimension "d65" = 20
  dimension "d68" = 20
  dimension "d69" = 20
  dimension "d72" = 370
  dimension "d73" = 0
  dimension "d76" = -370
  dimension "d77" = 0
  dimension "d80" = 0
  dimension "d81" = 400
  constraint tangent L0 A0
  constraint tangent A0 L1
  constraint parallel L0 L1
  constraint tangent L1 A1
  constraint tangent L0 A1
  constraint coincident P0 L4.start
  constraint midpoint L2 L4.end
  constraint perpendicular L2 L4
  constraint tangent L44 A28
  constraint tangent A29 L46
  constraint symmetric L4 L44.start A30.start
  constraint symmetric L4 A28.end L48.start
  constraint symmetric L4 L44.end L49.end
  constraint symmetric L4 L45.start L50.start
  constraint symmetric L4 A28 A31
  constraint symmetric L4 A29.start L48.end
  constraint symmetric L4 A29 A30
  constraint coincident L61.start A38.start
  constraint coincident A38.end L62.end
  constraint coincident A28.end L46.start
  measures "d52" distance of L2 L3
  measures "d56" radius of A1
  measures "d58" distance of A1.centre A0.centre
  measures "d64" distance of A28.centre L45.start
  measures "d65" radius of A29
  measures "d68" radius of A30
  measures "d69" radius of A31
extrude "Extrude2'" [suppressed] in component "SpoilBoard"
extrude "Extrude3" [suppressed] in component "SpoilBoard"
extrude "Extrude4" [suppressed] in component "SpoilBoard"
extrude "Extrude5" [suppressed] in component "SpoilBoard"
delete_face "DeleteFace1" [suppressed] in component "SpoilBoard"
delete_face "DeleteFace2" [suppressed] in component "SpoilBoard"
delete_face "DeleteFace3" [suppressed] in component "SpoilBoard"
delete_face "DeleteFace4" [suppressed] in component "SpoilBoard"
delete_face "DeleteFace5" [suppressed] in component "SpoilBoard"
delete_face "DeleteFace6" [suppressed] in component "SpoilBoard"
delete_face "DeleteFace7" [suppressed] in component "SpoilBoard"
delete_face "DeleteFace8" [suppressed] in component "SpoilBoard"
delete_face "DeleteFace9" [suppressed] in component "SpoilBoard"